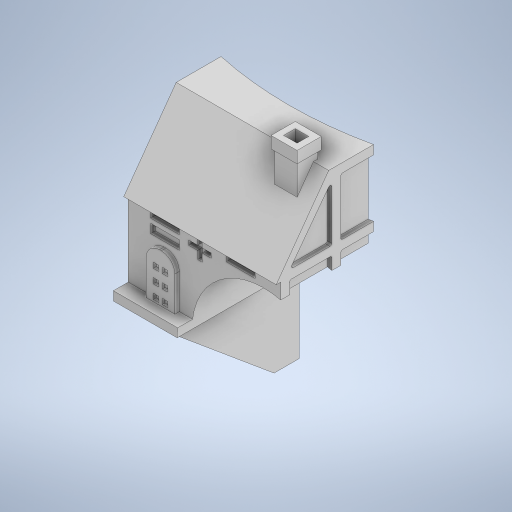
# Autodesk Inventor part: 屋2 物2
Saved by Autodesk Inventor 2024 (Build 280153000, 153)
## iProperties
Created: 2024-05-22
Part Number: 屋2 物2
Material: 一般
Document SubType Name: Modeling
Designer: User
Density: 1 g/cm^3
Appearance: 預設
Author: User
Autodesk Inventor part; units mm, degrees
ref_plane "YZ Plane" through (0, 0, 0) normal (1, 0, 0) x (0, 1, 0)
ref_plane "XZ Plane" through (0, 0, 0) normal (0, 1, 0) x (-1, 0, 0)
sketch "草圖1" plane through (0, 0, 0) normal (1, 0, 0) x (0, 1, 0)
  line L0 (0, 0) -> (0, 12)
  line L1 (0, 12) -> (1, 12)
  line L2 (1, 12) -> (1, 10.35)
  line L3 (1, 10.35) -> (9.5, 10.35)
  line L4 (9.5, 10.35) -> (9.5, 10.85)
  line L5 (9.5, 10.85) -> (17.6103, 5)
  line L6 (17.6103, 5) -> (17.6103, 0)
  line L7 (17.6103, 0) -> (0, 0)
  dimension "d0" = 12
  dimension "d1" = 1
  dimension "d2" = 1.65
  dimension "d3" = 8.5
  dimension "d4" = 0.5
  dimension "d5" = 10
  dimension "d6" = 5
  constraints: 16 end point, 5 perpendicular, 1 parallel, 1 vertical
  measures "d0" distance of L0.start L0.end
  measures "d1" distance of L0.end L1.end
  measures "d2" distance of L1.end L2.end
  measures "d3" distance of L2.end L3.end
  measures "d4" distance of L3.end L4.end
  measures "d5" distance of L4.end L5.end
  measures "d6" distance of L5.end L6.end
extrude "擠出1" add sketch "草圖1" along normal blind 17
sketch "草圖2" plane through (0, 0, 0) normal (-1, 0, 0) x (0, 0, 1)
  line L0 (0, 16.6103) -> (3.45, 16.6103)
  line L1 (3.65, 16.4103) -> (3.65, 10.4034)
  line L2 (3.45, 10.2034) -> (0, 10.2034)
  line L3 (0, 0) -> (0, 17.6103) projected
  line L4 (0, 9.2034) -> (3.45, 9.2034)
  line L5 (10.35, 1) -> (12, 1) projected
  line L6 (3.65, 9.0034) -> (3.65, 1.2)
  line L7 (4.65, 1.2) -> (4.65, 9.0034)
  line L8 (4.85, 9.2034) -> (9.15, 9.2034)
  line L9 (9.35, 9.0034) -> (9.35, 1.2)
  line L10 (4.65, 15.8842) -> (4.65, 10.4034)
  line L11 (4.85, 10.2034) -> (8.9506, 10.2034)
  line L12 (9.1107, 10.5232) -> (5.0101, 16.004)
  line L13 (9.15, 1) -> (4.85, 1)
  line L14 (3.45, 1) -> (0, 1)
  line L15 (0, 17.6103) -> (5, 17.6103) projected
  line L16 (5, 17.6103) -> (10.85, 9.5) projected
  line L17 (12, 0) -> (0, 0) projected
  line L18 (0, 16.6103) -> (0, 10.2034)
  line L19 (0, 9.2034) -> (0, 1)
  line L20 (10.35, 9.5) -> (10.35, 1) projected
  arc A0 (3.65, 16.4103) -> (3.45, 16.6103) centre (3.45, 16.4103) ccw
  arc A1 (5.0101, 16.004) -> (4.65, 15.8842) centre (4.85, 15.8842) ccw
  arc A2 (8.9506, 10.2034) -> (9.1107, 10.5232) centre (8.9506, 10.4034) ccw
  arc A3 (4.65, 10.4034) -> (4.85, 10.2034) centre (4.85, 10.4034) ccw
  arc A4 (3.45, 10.2034) -> (3.65, 10.4034) centre (3.45, 10.4034) ccw
  arc A5 (3.65, 9.0034) -> (3.45, 9.2034) centre (3.45, 9.0034) ccw
  arc A6 (3.45, 1) -> (3.65, 1.2) centre (3.45, 1.2) ccw
  arc A7 (9.15, 1) -> (9.35, 1.2) centre (9.15, 1.2) ccw
  arc A8 (9.35, 9.0034) -> (9.15, 9.2034) centre (9.15, 9.0034) ccw
  arc A9 (4.85, 9.2034) -> (4.65, 9.0034) centre (4.85, 9.0034) ccw
  arc A10 (4.65, 1.2) -> (4.85, 1) centre (4.85, 1.2) ccw
  point P0 (4.65, 16.4854)
  point P1 (4.65, 10.2034)
  point P2 (9.35, 10.2034)
  dimension "d10" = 1
  dimension "d11" = 1
  dimension "d12" = 1
  dimension "d13" = 1
  dimension "d14" = 1
  dimension "d15" = 1
  dimension "d16" = 1
  dimension "d17" = 1
  dimension "d18" = 1
  dimension "d19" = 4.7
  dimension "d20" = 0.2
  constraints: 30 end point, 22 point on circle, 22 tangent, 12 perpendicular, 11 centre point, 11 point on line, 10 equal radius, 2 collinear, 1 horizontal, 1 vertical
  measures "d10" distance between parallel lines of L15 L0
  measures "d11" angle of L16 L12
  measures "d12" distance between parallel lines of L17 L14
  measures "d13" distance between parallel lines of L17 L13
  measures "d14" distance between parallel lines of L20 L9
  measures "d15" distance between parallel lines of L6 L7
  measures "d16" distance between parallel lines of L1 L10
  measures "d17" distance between parallel lines of L2 L4
  measures "d18" distance between parallel lines of L11 L8
  measures "d19" distance between parallel lines of L9 L7
  measures "d20" radius of A0
extrude "擠出2" cut sketch "草圖2" against normal blind 0.5
ref_plane "工作平面1" through (8.5, 0, 0) normal (-1, 0, 0) x (0, 0, 1)
mirror "鏡射1" about plane through (8.5, 0, 0) normal (-1, 0, 0) of "擠出2"
sketch "草圖3" plane through (0, 0, 0) normal (0, -1, 0) x (1, 0, 0)
  line L0 (12.7976, 4.5211) -> (15.2976, 4.5211)
  line L1 (15.2976, 4.5211) -> (15.2976, 6.8211)
  line L2 (15.2976, 6.8211) -> (12.7976, 6.8211)
  line L3 (12.7976, 6.8211) -> (12.7976, 4.5211)
  point P0 (0, 0)
  dimension "d23" = 2.5
  dimension "d24" = 2.3
  constraints: 8 end point, 2 parallel, 1 horizontal, 1 perpendicular
  measures "d23" distance of L1.end L2.end
  measures "d24" distance of L0.end L1.end
extrude "擠出3" add sketch "草圖3" against normal blind 18.5
sketch "草圖4" plane through (0, 18.5, 0) normal (0, 1, 0) x (1, 0, 0)
  line L0 (12.5976, -4.3211) -> (15.4976, -4.3211)
  line L1 (15.4976, -4.3211) -> (15.4976, -7.0211)
  line L2 (15.4976, -7.0211) -> (12.5976, -7.0211)
  line L3 (12.5976, -7.0211) -> (12.5976, -4.3211)
  line L4 (15.2976, -4.5211) -> (12.7976, -4.5211) projected
  line L5 (15.2976, -6.8211) -> (15.2976, -4.5211) projected
  line L6 (12.7976, -4.5211) -> (12.7976, -6.8211) projected
  line L7 (12.7976, -6.8211) -> (15.2976, -6.8211) projected
  point P0 (0, 0)
  point P1 (15.2976, -5.4402)
  point P2 (12.7976, -5.4402)
  dimension "d27" = 0.2
  dimension "d28" = 0.2
  dimension "d29" = 0.2
  dimension "d30" = 0.2
  constraints: 8 end point, 2 parallel, 1 horizontal, 1 perpendicular
  measures "d27" distance between parallel lines of L4 L0
  measures "d28" distance between parallel lines of L1 L5
  measures "d29" distance between parallel lines of L6 L3
  measures "d30" distance between parallel lines of L2 L7
extrude "擠出4" add sketch "草圖4" along normal blind 1.3 contours L0 L1 L2 L3 | L5 L7 L6 L4
sketch "草圖5" plane through (0, 19.8, 0) normal (0, 1, 0) x (1, 0, 0)
  line L0 (14.7976, -5.0211) -> (13.2976, -5.0211)
  line L1 (13.2976, -5.0211) -> (13.2976, -6.3211)
  line L2 (13.2976, -6.3211) -> (14.7976, -6.3211)
  line L3 (14.7976, -6.3211) -> (14.7976, -5.0211)
  line L4 (15.4976, -7.0211) -> (15.4976, -4.3211) projected
  line L5 (12.5976, -7.0211) -> (15.4976, -7.0211) projected
  line L6 (12.5976, -4.3211) -> (12.5976, -7.0211) projected
  line L7 (15.4976, -4.3211) -> (12.5976, -4.3211) projected
  point P0 (0, 0)
  dimension "d33" = 0.7
  dimension "d34" = 0.7
  dimension "d35" = 0.7
  dimension "d36" = 0.7
  constraints: 8 end point, 2 parallel, 1 horizontal, 1 perpendicular
  measures "d33" distance between parallel lines of L4 L3
  measures "d34" distance between parallel lines of L5 L2
  measures "d35" distance between parallel lines of L6 L1
  measures "d36" distance between parallel lines of L7 L0
extrude "擠出5" cut sketch "草圖5" against normal blind 8 contours L3 L2 L1 L0
sketch "草圖6" plane through (0, 1, 10.35) normal (0, 0, 1) x (1, 0, 0)
  line L0 (2.5, 8.4383) -> (5.7, 8.4383)
  line L1 (5.7, 8.4383) -> (5.7, 7.4383)
  line L2 (5.7, 7.4383) -> (2.5, 7.4383)
  line L3 (2.5, 7.4383) -> (2.5, 8.4383)
  line L4 (0, 8.5) -> (0, 0) projected
  line L5 (2.5, 6.9383) -> (5.7, 6.9383)
  line L6 (5.7, 6.9383) -> (5.7, 5.9383)
  line L7 (5.7, 5.9383) -> (2.5, 5.9383)
  line L8 (2.5, 5.9383) -> (2.5, 6.9383)
  line L9 (9.2396, 7.4383) -> (9.2396, 6.9383)
  line L10 (6.7396, 6.9383) -> (6.7396, 7.4383)
  line L11 (7.7396, 8.0371) -> (8.2396, 8.0371)
  line L12 (8.2396, 6.0601) -> (7.7396, 6.0601)
  line L13 (6.7396, 7.4383) -> (7.7396, 7.4383)
  line L14 (8.2396, 7.4383) -> (9.2396, 7.4383)
  line L15 (7.7396, 6.0601) -> (7.7396, 6.9383)
  line L16 (7.7396, 7.4383) -> (7.7396, 8.0371)
  line L17 (8.2396, 8.0371) -> (8.2396, 7.4383)
  line L18 (8.2396, 6.9383) -> (8.2396, 6.0601)
  line L19 (9.2396, 6.9383) -> (8.2396, 6.9383)
  line L20 (7.7396, 6.9383) -> (6.7396, 6.9383)
  line L21 (10.9471, 8.4383) -> (14.1471, 8.4383)
  line L22 (14.1471, 8.4383) -> (14.1471, 7.4383)
  line L23 (14.1471, 7.4383) -> (10.9471, 7.4383)
  line L24 (10.9471, 7.4383) -> (10.9471, 8.4383)
  point P0 (0, -1)
  dimension "d39" = 3.2
  dimension "d40" = 1
  dimension "d41" = 2.5
  dimension "d42" = 3.2
  dimension "d43" = 1
  dimension "d44" = 0.5
  dimension "d45" = 2.5
  dimension "d46" = 2.5
  dimension "d49" = 3.2
  dimension "d50" = 1
  constraints: 48 end point, 16 parallel, 7 horizontal, 7 perpendicular, 1 collinear
  measures "d39" distance of L1.end L2.end
  measures "d40" distance of L0.end L1.end
  measures "d41" distance between parallel lines of L4 L3
  measures "d42" distance of L7.start L7.end
  measures "d43" distance of L5.end L7.start
  measures "d44" distance between parallel lines of L2 L5
  measures "d45" distance between parallel lines of L4 L8
  measures "d46" distance of L9.end L10.start
  measures "d49" distance of L23.start L23.end
  measures "d50" distance of L22.start L23.start
extrude "擠出6" cut sketch "草圖6" against normal blind 0.5
sketch "草圖7" plane through (0, 1, 10.35) normal (0, 0, 1) x (1, 0, 0)
  line L0 (2.5, 5.9383) -> (2.5, 6.9383) projected
  line L1 (2.5, 3.8861) -> (2.5, 0)
  line L2 (0, 0) -> (17, 0) projected
  line L3 (5.7, 6.9383) -> (5.7, 5.9383) projected
  line L4 (5.7, 3.8861) -> (5.7, 0)
  line L5 (4, 5.3861) -> (4.2, 5.3861)
  arc A0 (4, 5.3861) -> (2.5, 3.8861) centre (4, 3.8861) ccw
  arc A1 (5.7, 3.8861) -> (4.2, 5.3861) centre (4.2, 3.8861) ccw
  line L6 (4.1, 4.2144) -> (4.1, 0)
  line L7 (4.3, 0.2406) -> (4.9, 0.2406)
  line L8 (4.9, 0.2406) -> (4.9, 0.8406)
  line L9 (4.9, 0.8406) -> (4.3, 0.8406)
  line L10 (4.3, 0.8406) -> (4.3, 0.2406)
  line L11 (4.9, 2.3406) -> (4.3, 2.3406)
  line L12 (4.3, 2.3406) -> (4.3, 1.7406)
  line L13 (4.3, 1.7406) -> (4.9, 1.7406)
  line L14 (4.9, 1.7406) -> (4.9, 2.3406)
  line L15 (4.9, 3.8406) -> (4.3, 3.8406)
  line L16 (4.3, 3.8406) -> (4.3, 3.2406)
  line L17 (4.3, 3.2406) -> (4.9, 3.2406)
  line L18 (4.9, 3.2406) -> (4.9, 3.8406)
  line L19 (4.9, -6.1594) -> (4.3, -6.1594)
  line L20 (4.3, -6.1594) -> (4.3, -6.7594)
  line L21 (4.3, -6.7594) -> (4.9, -6.7594)
  line L22 (4.9, -6.7594) -> (4.9, -6.1594)
  line L23 (4.3, -7.6594) -> (4.3, -8.2594)
  line L24 (4.3, -8.2594) -> (4.9, -8.2594)
  line L25 (4.9, -8.2594) -> (4.9, -7.6594)
  line L26 (4.9, -7.6594) -> (4.3, -7.6594)
  line L27 (4.9, -9.1594) -> (4.3, -9.1594)
  line L28 (4.3, -9.1594) -> (4.3, -9.7594)
  line L29 (4.3, -9.7594) -> (4.9, -9.7594)
  line L30 (4.9, -9.7594) -> (4.9, -9.1594)
  line L31 (2.5, 0) -> (5.7, 0)
  line L32 (3.9, 3.8406) -> (3.3, 3.8406)
  line L33 (3.3, 3.8406) -> (3.3, 3.2406)
  line L34 (3.3, 3.2406) -> (3.9, 3.2406)
  line L35 (3.9, 3.2406) -> (3.9, 3.8406)
  line L36 (3.9, 2.3406) -> (3.3, 2.3406)
  line L37 (3.3, 2.3406) -> (3.3, 1.7406)
  line L38 (3.3, 1.7406) -> (3.9, 1.7406)
  line L39 (3.9, 1.7406) -> (3.9, 2.3406)
  line L40 (3.9, 0.8406) -> (3.3, 0.8406)
  line L41 (3.9, 0.2406) -> (3.9, 0.8406)
  line L42 (3.3, 0.2406) -> (3.9, 0.2406)
  line L43 (3.3, 0.8406) -> (3.3, 0.2406)
  point P0 (0, -1)
  point P1 (5.7, 0)
  dimension "d53" = 1.5
  dimension "d54" = 0.6
  dimension "d55" = 0.6
  dimension "d61" = 1.5
  dimension "d63" = 0.2
  dimension "d66" = 10
  dimension "d73" = 1
  constraints: 82 end point, 4 point on circle, 4 tangent, 4 vertical, 3 perpendicular, 2 centre point, 2 horizontal, 2 parallel, 2 point on line, 1 collinear, 1 equal radius, 64 other
  measures "d53" radius of A0
  measures "d54" distance of L9.end L8.end
  measures "d55" distance of L8.end L7.end
  measures "d61" distance of L8.end L11.start
  measures "d63" distance between parallel lines of L6 L10
  measures "d66" distance of L15.start L19.start
  measures "d73" distance of L15.start L32.start
extrude "擠出7" add sketch "草圖7" along normal blind 0.5 contours A0 L5 A1 L4 L2 L1
extrude "擠出8" add sketch "草圖7" along normal blind 0.2 contours L10 L9 L8 L7 | L14 L13 L12 L11 | L18 L17 L16 L15 | L35 L34 L33 L32 | L39 L38 L37 L36 | L41 L42 L43 L40
sketch "草圖8" plane through (0, 1, 10.35) normal (0, 0, 1) x (1, 0, 0)
  line L0 (5.7, 0) -> (17, 0) projected
  circle A0 centre (15.1042, -1) radius 8
  point P0 (0, -1)
  dimension "d83" = 16
  constraints: 1 centre point
  measures "d83" diameter of A0
extrude "擠出9" cut sketch "草圖8" along normal through all both and the other way through all
sketch "草圖9" plane through (0, 17.6103, 5) normal (0, 1, 0) x (1, 0, 0)
  line L0 (0, 5) -> (17, 5) projected
  arc A0 (0, 5) -> (17, 5) centre (8.5, 44.0864) ccw
  line L1 (0, 5) -> (17, 5)
  dimension "d86" = 40
  constraints: 2 end point, 2 point on circle, 1 centre point, 1 collinear
  measures "d86" radius of A0
extrude "擠出10" cut sketch "草圖9" against normal through all
sketch "草圖10" plane through (0, 0, 12) normal (0, -1, 0) x (1, 0, 0)
  line L0 (0, 0) -> (7.1042, 0) projected
  line L1 (0.7395, 0) -> (1.7395, 0)
  line L2 (1.7395, 0) -> (1.7395, -14.7929)
  line L3 (1.7395, -14.7929) -> (0.7395, -14.7929)
  line L4 (0.7395, -14.7929) -> (0.7395, 0)
  line L5 (2.9107, 0) -> (3.9107, 0)
  line L6 (3.9107, 0) -> (3.9107, -14.7929)
  line L7 (3.9107, -14.7929) -> (2.9107, -14.7929)
  line L8 (2.9107, -14.7929) -> (2.9107, 0)
  line L9 (4.9113, 0) -> (5.9113, 0)
  line L10 (5.9113, 0) -> (5.9113, -14.7929)
  line L11 (5.9113, -14.7929) -> (4.9113, -14.7929)
  line L12 (4.9113, -14.7929) -> (4.9113, 0)
  point P0 (0, -12)
  dimension "d89" = 1
  dimension "d90" = 1
  dimension "d91" = 1
  constraints: 24 end point, 6 parallel, 4 point on line, 3 horizontal, 3 perpendicular
  measures "d89" distance of L2.end L3.end
  measures "d90" distance of L6.end L7.end
  measures "d91" distance of L10.end L11.end
extrude "擠出11" add sketch "草圖10" along normal blind 10
sketch "草圖12" plane through (0.7395, 0, -2.7929) normal (-1, 0, 0) x (0, 0, 1)
  line L0 (14.7929, 0) -> (2.7929, 0) projected
  line L1 (14.7929, 0) -> (2.7929, -10)
  line L2 (14.7929, -10) -> (0, -10) projected
  line L3 (14.7929, 0) -> (14.7929, -10) projected
  line L4 (14.7929, -10) -> (14.7929, 0)
  line L5 (14.7929, -10) -> (2.7929, -10)
  constraints: 6 end point, 1 collinear, 1 perpendicular, 1 point on line
extrude "擠出13" cut sketch "草圖12" against normal up to surface (5.1718 mm away)
